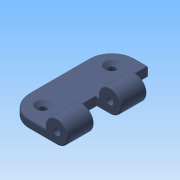
# Autodesk Inventor part: петля
Saved by Autodesk Inventor 2017 (Build 210142000, 142)
## iProperties
Part Number: петля
Material: Типовые
Document SubType Name: Modeling
Designer: Max
Mass: 4.48354 g
Surface Area: 29.6344 cm^2
Volume: 4.48354 cm^3
Density: 1 g/cm^3
Appearance: Резина — синяя
Author: Max
Autodesk Inventor part; units mm, degrees
ref_plane "YZ Plane" through (0, 0, 0) normal (1, 0, 0) x (0, 1, 0)
ref_plane "XZ Plane" through (0, 0, 0) normal (0, 1, 0) x (-1, 0, 0)
ref_plane "XY Plane" through (0, 0, 0) normal (0, 0, 1) x (1, 0, 0)
sketch "Эскиз1" plane through (0, 0, 0) normal (0, 0, 1) x (1, 0, 0)
  line L0 (-173.0013, 292.0364) -> (-157.0013, 292.0364)
  line L1 (-157.0013, 292.0364) -> (-157.0013, 246.0364)
  line L2 (-157.0013, 246.0364) -> (-173.0013, 246.0364)
  line L3 (-173.0013, 246.0364) -> (-173.0013, 292.0364)
  circle A0 centre (-165.0013, 284.0364) radius 1.5
  circle A1 centre (-165.0013, 254.0364) radius 1.5
  line L4 (-165.0013, 284.0364) -> (-165.0013, 254.0364) construction
  line L5 (-157.0013, 292.0364) -> (-145.0013, 292.0364)
  line L6 (-145.0013, 292.0364) -> (-145.0013, 280.5364)
  line L7 (-145.0013, 280.5364) -> (-157.0013, 280.5364) construction
  line L8 (-157.0013, 280.5364) -> (-157.0013, 292.0364)
  line L9 (-157.0013, 269.0364) -> (-145.0013, 269.0364) construction
  line L10 (-145.0013, 269.0364) -> (-145.0013, 257.5364)
  line L11 (-145.0013, 257.5364) -> (-157.0013, 257.5364) construction
  line L12 (-157.0013, 257.5364) -> (-157.0013, 269.0364)
  line L13 (-145.0013, 292.0364) -> (-129.0013, 292.0364)
  line L14 (-129.0013, 292.0364) -> (-129.0013, 246.0364)
  line L15 (-129.0013, 246.0364) -> (-145.0013, 246.0364)
  line L16 (-145.0013, 246.0364) -> (-145.0013, 292.0364)
  line L17 (-145.0013, 254.7807) -> (-145.0013, 246.0364)
  line L18 (-145.0013, 246.0364) -> (-157.0013, 246.0364)
  line L19 (-157.0013, 246.0364) -> (-157.0013, 254.7807)
  line L20 (-157.0013, 280.3864) -> (-145.0013, 280.3864)
  line L21 (-157.0013, 269.1864) -> (-145.0013, 269.1864)
  line L22 (-157.0013, 257.3864) -> (-145.0013, 257.3864)
  point P0 (0, 0)
  dimension "d0" = 3
  dimension "d1" = 3
  dimension "d2" = 8
  dimension "d3" = 8
  dimension "d4" = 30
  dimension "d5" = 46
  dimension "d6" = 8
  dimension "d7" = 8
  dimension "d8" = 46
  dimension "d9" = 16
  dimension "d10" = 44
  dimension "d11" = 12
  dimension "d12" = 16
  dimension "d13" = 11.5
  dimension "d14" = 11.5
  dimension "d15" = 11.5
  dimension "d16" = 11.5
  dimension "d17" = 0.15
  dimension "d18" = 0.15
  dimension "d19" = 0.15
  constraints: 46 end point, 9 parallel, 8 point on line, 7 perpendicular, 4 horizontal, 2 centre point, 1 midpoint, 1 vertical
  measures "d0" diameter of A0
  measures "d1" diameter of A1
  measures "d2" distance from line of L0 L4.start
  measures "d3" distance from line of L2 L4.end
  measures "d4" distance of L4.end L4.start
  measures "d5" distance between parallel lines of L2 L0
  measures "d6" distance between parallel lines of L1 L4
  measures "d7" distance between parallel lines of L4 L3
  measures "d8" distance between parallel lines of L15 L13
  measures "d9" distance between parallel lines of L16 L14
  measures "d10" distance between parallel lines of L14 L3
  measures "d11" distance between parallel lines of L6 L8
  measures "d12" distance between parallel lines of L3 L1
  measures "d13" distance between parallel lines of L7 L5
  measures "d14" distance between parallel lines of L9 L7
  measures "d15" distance between parallel lines of L11 L9
  measures "d16" distance between parallel lines of L18 L11
  measures "d17" distance between parallel lines of L22 L11
  measures "d18" distance between parallel lines of L9 L21
  measures "d19" distance between parallel lines of L7 L20
extrude "Выдавливание1" add sketch "Эскиз1" along normal blind 4 contours L0 L1 L2 L3
extrude "Выдавливание2" add sketch "Эскиз1" along normal blind 10 contours L1 L22 L16 L18 | L20 L16 L21 L1
sketch "Эскиз2" plane through (-173.0013, 246.0364, 0) normal (0, -1, 0) x (1, 0, 0)
  line L0 (28, 0) -> (16, 0) projected
  line L1 (22, 0) -> (22, 10) construction
  circle A0 centre (22, 5) radius 1.5
  line L2 (16, 10) -> (28, 10) projected
  circle A1 centre (22, 5) radius 5
  line L3 (28, 10) -> (16, 10) projected
  line L4 (22, 10) -> (28, 10)
  line L5 (28, 0) -> (28, 10) projected
  line L6 (28, 10) -> (28, 0)
  line L7 (28, 0) -> (22, 0)
  line L8 (16, 0) -> (28, 0) projected
  arc A2 (22, 0) -> (22, 10) centre (22, 5) ccw
  line L9 (0, 4) -> (16, 4) projected
  line L10 (16, 4) -> (17, 4)
  line L11 (17, 4) -> (17, 5)
  line L12 (16, 4) -> (16, 10) projected
  line L13 (16, 4) -> (16, 10)
  arc A3 (22, 10) -> (17, 5) centre (22, 5) ccw
  line L14 (16, 10) -> (22, 10)
  line L15 (16, 10) -> (28, 10) projected
  point P0 (173.0013, 0)
  dimension "d24" = 3
  constraints: 16 end point, 6 point on circle, 4 centre point, 4 collinear, 3 coincident, 3 midpoint, 3 tangent, 3 vertical, 1 perpendicular
  measures "d24" diameter of A0
extrude "Выдавливание3" cut sketch "Эскиз2" against normal blind 50 contours L0 A1 L2 L5 | L11 L10 L12 L2 A1
extrude "Выдавливание4" cut sketch "Эскиз2" against normal blind 50 contours A0
fillet "Сопряжение1" radius 10 2 edges at (-173.0013, 292.0364, 2) (-173.0013, 246.0364, 2)
fillet "Сопряжение2" radius 1 5 edges at (-160.0013, 292.0364, 4) (-173.0013, 269.0364, 4) (-170.0724, 248.9654, 4) (-159.5013, 246.0364, 4) (-170.0724, 289.1075, 4)
fillet "Сопряжение3" radius 0.5 24 edges at (-157.0013, 291.7435, 3.7071) (-157.0013, 292.0364, 1.5) (-157.0013, 285.7114, 4) (-154.0013, 280.3864, 0) (-156.0013, 280.3864, 4.5) (-147.4658, 280.3864, 8.5355) (-156.5013, 269.1864, 4) (-156.0013, 269.1864, 4.5) (-154.0013, 269.1864, 0) (-147.4658, 269.1864, 8.5355) (-157.0013, 263.2864, 4) (-156.5013, 257.3864, 4) (-154.0013, 257.3864, 0) (-156.0013, 257.3864, 4.5) (-147.4658, 257.3864, 8.5355) (-156.0013, 246.0364, 3.5) (-156.0013, 246.0364, 4.5) (-157.0013, 246.0364, 0) (-170.0724, 248.9654, 0) (-173.0013, 269.0364, 0) (-170.0724, 289.1075, 0) (-160.0013, 292.0364, 0) (-147.4658, 246.0364, 8.5355) (-156.5013, 280.3864, 4)
chamfer "Фаска1" distance 1.5 angle 45 2 edges at (-166.5013, 254.0364, 4) (-166.5013, 284.0364, 4)
